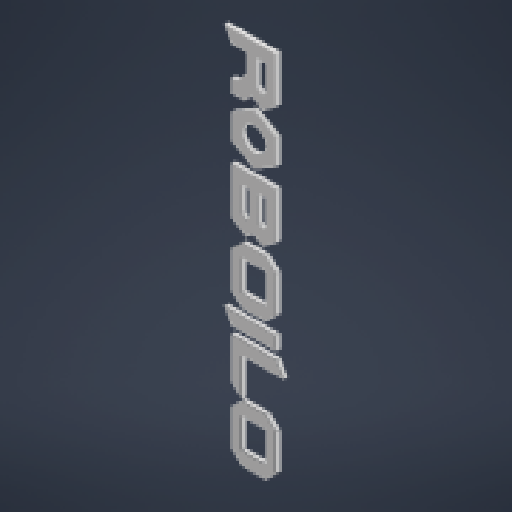
# Autodesk Inventor part: roboilo
Saved by Autodesk Inventor 2024 (Build 280153000, 153)
## iProperties
Created: 2024-06-09
Part Number: roboilo
Material: Generic
Document SubType Name: Modeling
Designer: mateu
Density: 1 g/cm^3
Appearance: Default
Author: mateu
Autodesk Inventor part; units mm, degrees
ref_plane "YZ Plane" through (0, 0, 0) normal (1, 0, 0) x (0, 1, 0)
ref_plane "XZ Plane" through (0, 0, 0) normal (0, 1, 0) x (-1, 0, 0)
ref_plane "XY Plane" through (0, 0, 0) normal (0, 0, 1) x (1, 0, 0)
sketch "Sketch1" plane through (0, 0, 0) normal (0, 0, 1) x (1, 0, 0)
  line L0 (13.187, 45.2611) -> (13.187, 52.8058)
  line L1 (11.8207, 44.2163) -> (13.187, 45.2611)
  line L2 (10.3841, 45.2712) -> (11.8207, 44.2163)
  line L3 (10.3841, 52.8058) -> (10.3841, 45.2712)
  line L4 (13.187, 52.8058) -> (10.3841, 52.8058)
  line L5 (3.0806, 40.1778) -> (3.0806, 44.1058)
  line L6 (6.8077, 40.1778) -> (3.0806, 40.1778)
  line L7 (9.0681, 42.4281) -> (6.8077, 40.1778)
  line L8 (12.0919, 40.1778) -> (9.0681, 42.4281)
  line L9 (16.0802, 43.1414) -> (12.0919, 40.1778)
  line L10 (16.0802, 56.7338) -> (16.0802, 43.1414)
  line L11 (0.8302, 56.7338) -> (16.0802, 56.7338)
  line L12 (3.0806, 52.8058) -> (0.8302, 56.7338)
  line L13 (7.4305, 52.8058) -> (3.0806, 52.8058)
  line L14 (7.4305, 47.3013) -> (7.4305, 52.8058)
  line L15 (4.3156, 44.1058) -> (7.4305, 47.3013)
  line L16 (3.0806, 44.1058) -> (4.3156, 44.1058)
  line L17 (3.0806, 27.8164) -> (3.0806, 35.3218)
  line L18 (9.5804, 24.0637) -> (3.0806, 27.8164)
  line L19 (16.0802, 27.8164) -> (9.5804, 24.0637)
  line L20 (16.0802, 35.3218) -> (16.0802, 27.8164)
  line L21 (9.5804, 39.0745) -> (16.0802, 35.3218)
  line L22 (3.0806, 35.3218) -> (9.5804, 39.0745)
  circle A0 centre (9.5804, 31.5691) radius 3.5
  line L23 (13.1669, 10.6183) -> (13.1669, 18.163)
  line L24 (12.0819, 9.664) -> (13.1669, 10.6183)
  line L25 (10.8965, 10.6183) -> (12.0819, 9.664)
  line L26 (10.8965, 18.163) -> (10.8965, 10.6183)
  line L27 (13.1669, 18.163) -> (10.8965, 18.163)
  line L28 (8.2443, 10.6183) -> (8.2443, 18.163)
  line L29 (7.0588, 9.664) -> (8.2443, 10.6183)
  line L30 (5.9739, 10.6183) -> (7.0588, 9.664)
  line L31 (5.9739, 18.163) -> (5.9739, 10.6183)
  line L32 (8.2443, 18.163) -> (5.9739, 18.163)
  line L33 (7.0588, 5.3642) -> (3.0605, 8.3178)
  line L34 (9.5704, 7.2127) -> (7.0588, 5.3642)
  line L35 (12.0819, 5.3642) -> (9.5704, 7.2127)
  line L36 (16.0802, 8.3178) -> (12.0819, 5.3642)
  line L37 (16.0802, 22.091) -> (16.0802, 8.3178)
  line L38 (3.0605, 22.091) -> (16.0802, 22.091)
  line L39 (3.0605, 8.3178) -> (3.0605, 22.091)
  line L40 (13.187, -9.5241) -> (13.187, -0.6233)
  line L41 (5.9739, -9.5241) -> (13.187, -9.5241)
  line L42 (5.9739, -0.6233) -> (5.9739, -9.5241)
  line L43 (13.187, -0.6233) -> (5.9739, -0.6233)
  line L44 (6.0341, -13.4521) -> (3.0806, -10.4986)
  line L45 (13.1267, -13.4521) -> (6.0341, -13.4521)
  line L46 (16.0802, -10.4986) -> (13.1267, -13.4521)
  line L47 (16.0802, 0.3512) -> (16.0802, -10.4986)
  line L48 (13.1267, 3.3048) -> (16.0802, 0.3512)
  line L49 (6.0341, 3.3048) -> (13.1267, 3.3048)
  line L50 (3.0806, 0.3512) -> (6.0341, 3.3048)
  line L51 (3.0806, -10.4986) -> (3.0806, 0.3512)
  line L52 (3.0605, -19.4798) -> (0.8302, -15.5518)
  line L53 (16.0802, -19.4798) -> (3.0605, -19.4798)
  line L54 (16.0802, -15.5518) -> (16.0802, -19.4798)
  line L55 (0.8302, -15.5518) -> (16.0802, -15.5518)
  line L56 (5.9739, -36.8094) -> (3.0605, -33.896)
  line L57 (5.9739, -25.6381) -> (5.9739, -36.8094)
  line L58 (18.3607, -25.6381) -> (5.9739, -25.6381)
  line L59 (16.0903, -21.7101) -> (18.3607, -25.6381)
  line L60 (3.0605, -21.7101) -> (16.0903, -21.7101)
  line L61 (3.0605, -33.896) -> (3.0605, -21.7101)
  line L62 (13.187, -50.0803) -> (13.187, -41.1794)
  line L63 (5.9739, -50.0803) -> (13.187, -50.0803)
  line L64 (5.9739, -41.1794) -> (5.9739, -50.0803)
  line L65 (13.187, -41.1794) -> (5.9739, -41.1794)
  line L66 (6.0341, -54.0083) -> (3.0806, -51.0548)
  line L67 (13.1267, -54.0083) -> (6.0341, -54.0083)
  line L68 (16.0802, -51.0548) -> (13.1267, -54.0083)
  line L69 (16.0802, -40.2049) -> (16.0802, -51.0548)
  line L70 (13.1267, -37.2514) -> (16.0802, -40.2049)
  line L71 (6.0341, -37.2514) -> (13.1267, -37.2514)
  line L72 (3.0806, -40.2049) -> (6.0341, -37.2514)
  line L73 (3.0806, -51.0548) -> (3.0806, -40.2049)
  point P0 (0, 0)
extrude "Extrusion1" add sketch "Sketch1" along normal blind 1.2
body "Solid1"
